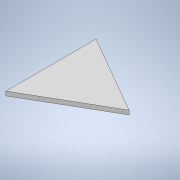
# Autodesk Inventor part: objeto2
Saved by Autodesk Inventor 2022.3 (Build 263350000, 350)
## iProperties
Created: 2023-06-18
Part Number: objeto2
Material: Generic
Document SubType Name: Modeling
Designer: crist
Density: 1 g/cm^3
Appearance: Default
Author: crist
Autodesk Inventor part; units mm, degrees
ref_plane "YZ Plane" through (0, 0, 0) normal (1, 0, 0) x (0, 1, 0)
ref_plane "XZ Plane" through (0, 0, 0) normal (0, 1, 0) x (-1, 0, 0)
ref_plane "XY Plane" through (0, 0, 0) normal (0, 0, 1) x (1, 0, 0)
sketch "Sketch1" plane through (0, 0, 0) normal (0, 1, 0) x (-1, 0, 0)
  line L0 (25, -43.3013) -> (-50, 0)
  line L1 (-50, 0) -> (25, 43.3013)
  line L2 (25, 43.3013) -> (25, -43.3013)
  circle A0 centre (0, 0) radius 25 construction
  point P0 (25, 0)
  constraints: 6 end point, 1 centre point, 1 coincident, 1 midpoint, 1 tangent, 7 other
extrude "Extrusion1" add sketch "Sketch1" along normal blind 4
body "Solid1"
